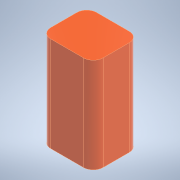
# Autodesk Inventor part: AA-Cellx4
Saved by Autodesk Inventor 2022 (Build 260153000, 153)
## iProperties
Created: 2024-07-05
Part Number: AA-Cellx4
Material: 一般
Document SubType Name: Modeling
Designer: yamashita1
Density: 1 g/cm^3
Appearance: 滑らか - 淡いオレンジ
Author: yamashita1
Autodesk Inventor part; units mm, degrees
ref_plane "YZ Plane" through (0, 0, 0) normal (1, 0, 0) x (0, 1, 0)
ref_plane "XZ Plane" through (0, 0, 0) normal (0, 1, 0) x (-1, 0, 0)
ref_plane "XY Plane" through (0, 0, 0) normal (0, 0, 1) x (1, 0, 0)
sketch "スケッチ1" plane through (0, 0, 0) normal (0, 0, 1) x (1, 0, 0)
  line L0 (-16, 29) -> (16, 29)
  line L1 (16, 29) -> (16, -29)
  line L2 (16, -29) -> (-16, -29)
  line L3 (-16, -29) -> (-16, 29)
  point P0 (0, 0)
  point P1 (-16, 0)
  point P2 (0, -29)
  dimension "d0" = 32
  dimension "d1" = 58
  constraints: 8 end point, 2 midpoint, 2 parallel, 1 horizontal, 1 horizontal alignment, 1 perpendicular, 1 vertical alignment
  measures "d0" distance of L1.end L2.end
  measures "d1" distance of L0.end L1.end
extrude "押し出し1" add sketch "スケッチ1" along normal blind 28
fillet "フィレット1" radius 6 4 edges at (16, 0, 28) (-16, 0, 28) (-16, 0, 0) (16, 0, 0)
